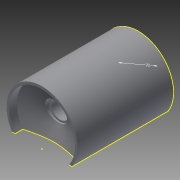
# Autodesk Inventor part: obudowa - klosz dla zarowki v2,2
Saved by Autodesk Inventor 2014 (Build 180170000, 170)
## iProperties
Created: 2018-02-27
Part Number: obudowa - klosz dla zarowki v2,2
Material: Generic
Document SubType Name: Modeling
Designer: HP820
Density: 1 g/cm^3
Appearance: Default
Author: HP820
Autodesk Inventor part; units mm, degrees
ref_plane "YZ Plane" through (0, 0, 0) normal (1, 0, 0) x (0, 1, 0)
ref_plane "XZ Plane" through (0, 0, 0) normal (0, 1, 0) x (-1, 0, 0)
ref_plane "XY Plane" through (0, 0, 0) normal (0, 0, 1) x (1, 0, 0)
sketch "Sketch1" plane through (0, 0, 0) normal (0, 1, 0) x (-1, 0, 0)
  line L0 (-45, 0) -> (45, 0)
  arc A0 (45, 0) -> (-45, 0) centre (0, 31.6228) ccw
  line L1 (-45, 0) -> (-50, 0)
  line L2 (45, 0) -> (50, 0)
  arc A1 (50, 0) -> (-50, 0) centre (0, 31.6228) ccw
  point P0 (0, 0)
  dimension "d0" = 90
  dimension "d1" = 45
  dimension "d2" = 55
  dimension "d3" = 5
  dimension "d4" = 5
  constraints: 6 end point, 4 point on circle, 2 centre point, 2 collinear, 1 horizontal
  measures "d0" distance of L0.start L0.end
  measures "d1" distance of L0.start point (0, 0)
  measures "d2" radius of A0
  measures "d3" distance of L0.start L1.end
  measures "d4" distance of L0.end L2.end
extrude "Extrusion1" add sketch "Sketch1" along normal blind 160 contours L1 A1 L2 A0
sketch "Sketch2" plane through (0, 160, 0) normal (0, 1, 0) x (1, 0, 0)
  arc A0 (-45, 0) -> (45, 0) centre (0, -31.6228) ccw projected
  line L0 (-45, 0) -> (-50, 0) projected
  arc A1 (-50, 0) -> (50, 0) centre (0, -31.6228) ccw projected
  line L1 (50, 0) -> (45, 0) projected
  circle A2 centre (0, -42.471) radius 35
  point P0 (0, 0)
  dimension "d7" = 70
  constraints: 1 centre point
  measures "d7" diameter of A2
ref_plane "Work Plane1" through (0, 30, 0) normal (0, -1, 0) x (1, 0, 0)
sketch "Sketch3" plane through (0, 30, 0) normal (0, -1, 0) x (1, 0, 0)
  arc A0 (45, 0) -> (-45, 0) centre (0, 31.6228) ccw projected
  line L0 (50, 0) -> (45, 0) projected
  arc A1 (50, 0) -> (-50, 0) centre (0, 31.6228) ccw projected
  line L1 (-45, 0) -> (-50, 0) projected
  line L2 (-45, 0) -> (45, 0)
  point P0 (0, 0)
  constraints: 2 end point, 1 collinear
extrude "Extrusion2" add sketch "Sketch3" against normal blind 19 contours L2 A0
chamfer "Chamfer1" distance 55 distance2 17 1 edges at (0, 30, 86.6228) measured on face at (0, 30, 86.1228)
sketch "Sketch4" plane through (-50, 0, 0) normal (0, 0, -1) x (-1, 0, 0)
  line L0 (-100, 0) -> (-95, 0) projected
  line L1 (-95, 0) -> (-95, 13) projected
  line L2 (-5, 0) -> (-5, 13) projected
  line L3 (-5, 0) -> (0, 0) projected
  line L4 (0, 0) -> (0, 160) projected
  line L5 (-5, 160) -> (0, 160) projected
  line L6 (-5, 49) -> (-5, 160) projected
  line L7 (-95, 49) -> (-5, 49) projected
  line L8 (-95, 49) -> (-95, 160) projected
  line L9 (-100, 160) -> (-95, 160) projected
  line L10 (-100, 0) -> (-100, 160) projected
  point P0 (-50, 0)
  constraints: 1 horizontal alignment
sketch "Sketch5" plane through (0, 49, 0) normal (0, 1, 0) x (1, 0, 0)
  circle A0 centre (0, -42.4934) radius 16.5
  dimension "d14" = 33
  constraints: 1 centre point
  measures "d14" diameter of A0
ref_plane "Work Plane2" through (0, 30, 0) normal (0, 1, 0) x (1, 0, 0)
sketch "Sketch6" plane through (0, 30, 0) normal (0, 1, 0) x (1, 0, 0)
  circle A0 centre (0, -42.4886) radius 18
  point P0 (0, 0)
  dimension "d16" = 36
  constraints: 1 centre point
  measures "d16" diameter of A0
extrude "Extrusion3" cut sketch "Sketch6" against normal blind 27
sketch "Sketch7" plane through (0, 30, 0) normal (0, 1, 0) x (1, 0, 0)
  circle A0 centre (0, -42.5113) radius 15
  point P0 (0, 0)
  dimension "d19" = 30
  constraints: 1 centre point
  measures "d19" diameter of A0
loft "Loft1" cut profiles "Sketch7", "Sketch5"
equation "\"d1\" = 0.5 * d0"
body "Solid1"
